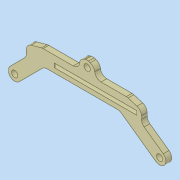
# Autodesk Inventor part: ArduinoMegaHolder1
Saved by Autodesk Inventor 2017 (Build 210142000, 142)
## iProperties
Created: 2017-04-22
Part Number: ArduinoMegaHolder1
Material: ABS Plastic
Document SubType Name: Modeling
Designer: Derek Wider
Mass: 1.76752 g
Surface Area: 21.643 cm^2
Volume: 1.66747 cm^3
Density: 1.06 g/cm^3
Appearance: Smooth - Ash
Author: Derek Wider
Autodesk Inventor part; units mm, degrees
ref_plane "YZ Plane" through (0, 0, 0) normal (1, 0, 0) x (0, 1, 0)
ref_plane "XZ Plane" through (0, 0, 0) normal (0, 1, 0) x (-1, 0, 0)
ref_plane "XY Plane" through (0, 0, 0) normal (0, 0, 1) x (1, 0, 0)
sketch "Sketch1" plane through (0, 0, 0) normal (0, 0, 1) x (1, 0, 0)
  circle A0 centre (0, 0) radius 1.5875
  circle A1 centre (0, 0) radius 3.175
  line L0 (0, 0) -> (36.2951, -20.955)
  line L1 (0, 0) -> (41.91, 0) construction
  circle A2 centre (36.2951, -20.955) radius 1.5875
  circle A3 centre (36.2951, -20.955) radius 3.175
  line L2 (0, 0) -> (0, 8.5417)
  circle A4 centre (-36.2951, -20.955) radius 1.5875
  circle A5 centre (-36.2951, -20.955) radius 3.175
  line L3 (-29.1831, -8.3058) -> (24.9189, -8.3058)
  line L4 (24.9189, -8.3058) -> (24.9189, -6.2738)
  line L5 (24.9189, -6.2738) -> (-29.1831, -6.2738)
  line L6 (-29.1831, -6.2738) -> (-29.1831, -8.3058)
  line L7 (-16.4831, -6.2738) -> (-16.4831, -8.3058)
  line L8 (-30.4531, -5.0038) -> (27.2049, -5.0038)
  line L9 (27.2049, -5.0038) -> (27.2049, -10.5918)
  line L10 (27.2049, -10.5918) -> (-30.4531, -10.5918)
  line L11 (-30.4531, -10.5918) -> (-30.4531, -5.0038)
  line L12 (-30.4531, -5.0038) -> (-0.8344, 3.0634)
  line L13 (-30.4531, -10.5918) -> (-38.5445, -18.7142)
  line L14 (27.2049, -5.0038) -> (0.6506, 3.1076)
  line L15 (27.2049, -10.5918) -> (38.1356, -18.3679)
  line L16 (34.4546, -23.5421) -> (16.2505, -10.5918)
  line L17 (-34.0458, -23.1958) -> (-21.49, -10.5918)
  dimension "d0" = 3.175
  dimension "d1" = 6.35
  dimension "d2" = 41.91
  dimension "d3" = 30
  dimension "d4" = 3.175
  dimension "d5" = 6.35
  dimension "d6" = 7.112
  dimension "d7" = 12.6492
  dimension "d8" = 54.102
  dimension "d9" = 41.402
  dimension "d10" = 1.27
  dimension "d11" = 2.286
  dimension "d12" = 1.27
  dimension "d13" = 2.286
  dimension "d16" = 2.032
  constraints: 36 end point, 6 centre point, 6 parallel, 6 point on circle, 5 coincident, 5 tangent, 4 point on line, 3 horizontal, 3 perpendicular, 2 symmetric about line, 1 equal length, 1 vertical, 2 other
  measures "d0" diameter of A0
  measures "d1" diameter of A1
  measures "d2" distance of L0.start L0.end
  measures "d3" angle of L0 L1
  measures "d4" diameter of A2
  measures "d5" diameter of A3
  measures "d6" horizontal distance of L3.start A4.centre
  measures "d7" vertical distance of A4.centre L3.start
  measures "d8" distance of L4.end L5.end
  measures "d9" distance between parallel lines of L4 L7
  measures "d10" distance between parallel lines of L8 L5
  measures "d11" distance between parallel lines of L3 L10
  measures "d12" distance between parallel lines of L6 L11
  measures "d13" distance between parallel lines of L4 L9
  measures "d16" distance between parallel lines of L5 L3
extrude "Extrusion1" add sketch "Sketch1" along normal blind 2.8575 contours A0 L2 A1 L14 L0 | A0 L0 A1 L2 | L0 L8 L12 A1 | A1 L14 L8 L0 | L8 L9 L10 L0 L3 L4 L5 | L0 L5 L6 L3 L10 L11 L8 | L10 L17 A5 L13 | L15 A3 L0 L10 | A5 | L0 A3 L16 L10 | A3
fillet "Fillet1" radius 3.175 6 edges at (27.2049, -10.5918, 1.4287) (27.2049, -5.0038, 1.4287) (-30.4531, -5.0038, 1.4287) (-30.4531, -10.5918, 1.4287) (-21.49, -10.5918, 1.4287) (16.2505, -10.5918, 1.4287)
sketch "Sketch4" plane through (0, 0, 0) normal (0, 0, -1) x (-1, 0, 0)
  arc A0 (30.4531, -7.4297) -> (28.1125, -4.3663) centre (27.2781, -7.4297) ccw projected
  line L0 (0.8344, 3.0634) -> (28.1125, -4.3663) projected
  arc A1 (0.8344, 3.0634) -> (-0.6506, 3.1076) centre (0, 0) ccw projected
  line L1 (-24.9574, -4.3173) -> (-0.6506, 3.1076) projected
  arc A2 (-24.9574, -4.3173) -> (-27.2049, -7.3538) centre (-24.0299, -7.3538) ccw projected
  line L2 (-27.2049, -8.954) -> (-27.2049, -7.3538) projected
  arc A3 (-28.5394, -11.5412) -> (-27.2049, -8.954) centre (-30.3799, -8.954) ccw projected
  line L3 (-38.1356, -18.3679) -> (-28.5394, -11.5412) projected
  arc A4 (-38.1356, -18.3679) -> (-34.4546, -23.5421) centre (-36.2951, -20.955) ccw projected
  line L4 (-17.0769, -11.1797) -> (-34.4546, -23.5421) projected
  arc A5 (-15.2364, -10.5918) -> (-17.0769, -11.1797) centre (-15.2364, -13.7668) ccw projected
  line L5 (20.1713, -10.5918) -> (-15.2364, -10.5918) projected
  arc A6 (22.4207, -11.526) -> (20.1713, -10.5918) centre (20.1713, -13.7668) ccw projected
  line L6 (34.0458, -23.1958) -> (22.4207, -11.526) projected
  arc A7 (34.0458, -23.1958) -> (38.5445, -18.7142) centre (36.2951, -20.955) ccw projected
  line L7 (31.3788, -11.521) -> (38.5445, -18.7142) projected
  arc A8 (30.4531, -9.2802) -> (31.3788, -11.521) centre (33.6281, -9.2802) ccw projected
  line L8 (30.4531, -7.4297) -> (30.4531, -9.2802) projected
  circle A9 centre (36.2951, -20.955) radius 1.5875 projected
  line L9 (29.1831, -8.3058) -> (-24.9189, -8.3058) projected
  line L10 (-24.9189, -8.3058) -> (-24.9189, -6.2738) projected
  line L11 (-24.9189, -6.2738) -> (29.1831, -6.2738) projected
  line L12 (29.1831, -6.2738) -> (29.1831, -8.3058) projected
  circle A10 centre (0, 0) radius 1.5875 projected
  circle A11 centre (-36.2951, -20.955) radius 1.5875 projected
  line L13 (-23.2186, 2.3851) -> (-3.81, 2.3851)
  line L14 (-3.81, 2.3851) -> (-3.81, -2.8268)
  line L15 (-3.81, -2.8268) -> (-23.2186, -2.8268)
  line L16 (-23.2186, -2.8268) -> (-23.2186, 2.3851)
  line L17 (23.7839, 2.3851) -> (3.81, 2.3851)
  line L18 (3.81, 2.3851) -> (3.81, -2.8268)
  line L19 (3.81, -2.8268) -> (23.7839, -2.8268)
  line L20 (23.7839, -2.8268) -> (23.7839, 2.3851)
  dimension "d23" = 3.81
  dimension "d24" = 3.81
  constraints: 16 end point, 4 parallel, 2 horizontal, 2 perpendicular, 2 point on line
  measures "d23" distance from line of point (0, 0) L14
  measures "d24" distance from line of L18 point (0, 0)
extrude "Extrusion3" cut sketch "Sketch4" against normal through all contours L19 L18 L0 | L0 L18 L17 L20 L19 | L14 L15 L1 | L1 L15 L16 L13 L14
fillet "Fillet2" radius 3.175 6 edges at (3.81, 2.1425, 1.4287) (3.81, -2.8268, 1.4287) (-3.81, -2.8268, 1.4287) (-3.81, 2.2529, 1.4287) (20.0782, -2.8268, 1.4287) (-22.4604, -2.8268, 1.4287)
sketch "Sketch7" plane through (0, 0, 2.8575) normal (0, 0, 1) x (1, 0, 0)
  line L0 (-16.4831, -6.2738) -> (-16.4831, -8.3058) projected
  line L1 (-29.1831, -8.3058) -> (-29.1831, -6.2738) projected
  line L2 (-16.4831, -8.3058) -> (-29.1831, -8.3058)
  line L3 (-29.1831, -8.3058) -> (-29.1831, -6.2738)
  line L4 (-29.1831, -6.2738) -> (-16.4831, -6.2738)
  line L5 (-16.4831, -6.2738) -> (-16.4831, -8.3058)
  point P0 (0, 0)
  constraints: 8 end point, 2 parallel, 1 horizontal, 1 perpendicular
extrude "Extrusion5" add sketch "Sketch7" against normal blind 0.508
body "Solid1"
